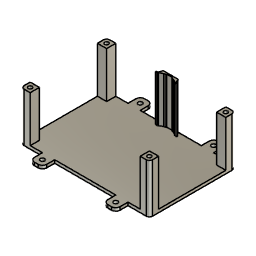
din_shelf_mount_2 v2 (Autodesk Fusion 360 design; units mm, degrees)
Autodesk Fusion 360 part; units mm, degrees
sketch "Sketch1" plane through (0, 0, 0) normal (0, 0, 1) x (1, 0, 0)
  line L0 (0, 0) -> (210, 0)
  line L1 (210, 0) -> (210, 140)
  line L2 (210, 140) -> (0, 140)
  line L3 (0, 140) -> (0, 0)
  line L4 (35, 140) -> (55, 140)
  line L5 (55, 140) -> (55, 153)
  line L6 (48, 160) -> (42, 160)
  line L7 (35, 153) -> (35, 140)
  line L8 (0, 70) -> (210, 70)
  line L9 (105, 140) -> (105, 0)
  circle A0 centre (45, 150) radius 3.5
  arc A1 (42, 160) -> (35, 153) centre (42, 153) ccw
  arc A2 (55, 153) -> (48, 160) centre (48, 153) ccw
  arc A3 (35, -13) -> (42, -20) centre (42, -13) ccw
  line L10 (48, -20) -> (42, -20)
  circle A4 centre (45, -10) radius 3.5
  arc A5 (48, -20) -> (55, -13) centre (48, -13) ccw
  line L11 (35, -13) -> (35, 0)
  line L12 (55, 0) -> (55, -13)
  arc A6 (162, 160) -> (155, 153) centre (162, 153) ccw
  arc A7 (175, 153) -> (168, 160) centre (168, 153) ccw
  line L13 (162, 160) -> (168, 160)
  circle A8 centre (165, 150) radius 3.5
  line L14 (175, 153) -> (175, 140)
  line L15 (155, 140) -> (155, 153)
  arc A9 (155, -13) -> (162, -20) centre (162, -13) ccw
  circle A10 centre (165, -10) radius 3.5
  line L16 (162, -20) -> (168, -20)
  arc A11 (168, -20) -> (175, -13) centre (168, -13) ccw
  line L17 (155, 0) -> (155, -13)
  line L18 (175, -13) -> (175, 0)
  point P0 (35, 160)
  point P1 (35, -20)
  point P2 (175, 160)
  point P3 (175, -20)
  dimension "d1" = 210
  dimension "d2" = 140
  dimension "d3" = 20
  dimension "d4" = 20
  dimension "d5" = 35
  dimension "d6" = 7
  dimension "d7" = 10
  dimension "d8" = 10
  dimension "d9" = 7
  constraint horizontal L0
  constraint vertical L1
  constraint horizontal L2
  constraint vertical L3
  constraint coincident L0.start L3.end
  constraint horizontal L4
  constraint vertical L5
  constraint horizontal L6
  constraint vertical L7
  constraint coincident L2 L4.start
  constraint midpoint L3 L8.start
  constraint midpoint L1 L8.end
  constraint midpoint L2 L9.start
  constraint midpoint L0 L9.end
  constraint coincident P0 L6
  constraint coincident P0 L7
  constraint tangent L6 A1
  constraint tangent L7 A1
  constraint tangent L5 A2
  constraint tangent L6 A2
  constraint equal A1 A2
  constraint symmetric L4.start L8 L11.end
  constraint symmetric L4.end L8 L12.start
  constraint symmetric P0 L8 P1
  constraint symmetric L8 A0 A4
  constraint symmetric L8 L6.end A3.end
  constraint symmetric L8 L7.start A3.start
  constraint symmetric L8 A1 A3
  constraint symmetric L8 L5.end A5.end
  constraint symmetric L8 L6.start L10.start
  constraint symmetric L8 A2 A5
  constraint symmetric L4.start L9 L14.end
  constraint symmetric L4.end L9 L15.start
  constraint symmetric P0 L9 P2
  constraint symmetric L9 A0 A8
  constraint symmetric L9 L6.end A7.end
  constraint symmetric L9 L7.start A7.start
  constraint symmetric L9 A1 A7
  constraint symmetric L9 L5.end A6.end
  constraint symmetric L9 L6.start A6.start
  constraint symmetric L9 A2 A6
  constraint symmetric L9 A3.start A11.end
  constraint symmetric L9 P1 P3
  constraint symmetric L9 L10.start A9.end
  constraint symmetric L9 A5.end A9.start
  constraint symmetric L9 A3.end L16.end
  constraint symmetric L9 A3 A11
  constraint symmetric L9 A4 A10
  constraint symmetric L9 A5 A9
  constraint symmetric L9 L11.end L18.end
  constraint symmetric L9 L12.start L17.start
  measures "d1" distance of L0.start L0.end
  measures "d2" distance of L0.start L2.end
  measures "d3" distance of L4.start L4.end
  measures "d4" distance of L4.start P0
  measures "d5" distance of L3 L7
  measures "d6" diameter of A0
  measures "d7" distance of L6 A0.centre
  measures "d8" distance of L7 A0.centre
  measures "d9" radius of A1
extrude "Extrude1" add sketch "Sketch1" along normal blind 5 makes body 1
sketch "Sketch2" plane through (0, 0, 5) normal (0, 0, 1) x (-1, 0, 0)
  circle A0 centre (-45, 10) radius 3.5
  circle A1 centre (-45, -150) radius 3.5
  circle A2 centre (-165, -150) radius 3.5
  circle A3 centre (-165, 10) radius 3.5
  line L0 (-55, 0) -> (-155, 0)
  line L1 (-155, 0) -> (-155, 13)
  arc A4 (-155, 13) -> (-162, 20) centre (-162, 13) ccw
  line L2 (-162, 20) -> (-168, 20)
  arc A5 (-168, 20) -> (-175, 13) centre (-168, 13) ccw
  line L3 (-175, 13) -> (-175, 0)
  line L4 (-175, 0) -> (-210, 0)
  line L5 (-210, 0) -> (-210, -140)
  line L6 (-210, -140) -> (-175, -140)
  line L7 (-175, -140) -> (-175, -153)
  arc A6 (-175, -153) -> (-168, -160) centre (-168, -153) ccw
  line L8 (-168, -160) -> (-162, -160)
  arc A7 (-162, -160) -> (-155, -153) centre (-162, -153) ccw
  line L9 (-155, -153) -> (-155, -140)
  line L10 (-155, -140) -> (-55, -140)
  line L11 (-55, -140) -> (-55, -153)
  arc A8 (-55, -153) -> (-48, -160) centre (-48, -153) ccw
  line L12 (-48, -160) -> (-42, -160)
  arc A9 (-42, -160) -> (-35, -153) centre (-42, -153) ccw
  line L13 (-35, -153) -> (-35, -140)
  line L14 (-35, -140) -> (0, -140)
  line L15 (0, -140) -> (0, 0)
  line L16 (0, 0) -> (-35, 0)
  line L17 (-35, 0) -> (-35, 13)
  arc A10 (-35, 13) -> (-42, 20) centre (-42, 13) ccw
  line L18 (-42, 20) -> (-48, 20)
  arc A11 (-48, 20) -> (-55, 13) centre (-48, 13) ccw
  line L19 (-55, 13) -> (-55, 0)
  line L20 (0, -140) -> (-15, -140)
  line L21 (-15, -140) -> (-15, -125)
  line L22 (-15, -125) -> (0, -125)
  line L23 (0, -125) -> (0, -140)
  line L24 (-210, -140) -> (-195, -140)
  line L25 (-195, -140) -> (-195, -125)
  line L26 (-195, -125) -> (-210, -125)
  line L27 (-210, -125) -> (-210, -140)
  line L28 (0, 0) -> (-15, 0)
  line L29 (-15, 0) -> (-15, -15)
  line L30 (-15, -15) -> (0, -15)
  line L31 (0, -15) -> (0, 0)
  line L32 (-210, 0) -> (-195, 0)
  line L33 (-195, 0) -> (-195, -15)
  line L34 (-195, -15) -> (-210, -15)
  line L35 (-210, -15) -> (-210, 0)
  dimension "d12" = 15
  dimension "d13" = 15
  dimension "d14" = 15
  dimension "d15" = 15
  dimension "d16" = 15
  dimension "d17" = 15
  dimension "d18" = 15
  dimension "d19" = 15
  constraint horizontal L20
  constraint vertical L21
  constraint horizontal L22
  constraint vertical L23
  constraint coincident L14.end L15.start
  constraint horizontal L24
  constraint vertical L25
  constraint horizontal L26
  constraint vertical L27
  constraint coincident L5.end L6.start
  constraint horizontal L28
  constraint vertical L29
  constraint horizontal L30
  constraint vertical L31
  constraint coincident L15.end L16.start
  constraint horizontal L32
  constraint vertical L33
  constraint horizontal L34
  constraint vertical L35
  constraint coincident L4.end L5.start
  measures "d12" distance of L14.end L20.end
  measures "d13" distance of L14.end L22.end
  measures "d14" distance of L5.end L24.end
  measures "d15" distance of L5.end L26.end
  measures "d16" distance of L15.end L28.end
  measures "d17" distance of L15.end L30.end
  measures "d18" distance of L4.end L32.end
  measures "d19" distance of L4.end L34.end
extrude "Extrude2" add sketch "Sketch2" along normal blind 75 contours L15 L16 L28 L29 L30 L31 | L4 L5 L32 L33 L34 L35 | L14 L15 L20 L21 L22 L23 | L5 L6 L24 L25 L26 L27 bodies 1
fillet "Fillet1" radius 5 4 edges at (0, 140, 40) (0, 0, 40) (210, 140, 40) (210, 0, 40) on bodies 1
sketch "Sketch3" plane through (0, 0, 5) normal (0, 0, 1) x (-1, 0, 0)
  line L0 (-15, -15) -> (-15, 0)
  line L1 (-15, 0) -> (-35, 0)
  line L2 (-35, 0) -> (-35, 13)
  arc A0 (-35, 13) -> (-42, 20) centre (-42, 13) ccw
  line L3 (-42, 20) -> (-48, 20)
  arc A1 (-48, 20) -> (-55, 13) centre (-48, 13) ccw
  line L4 (-55, 13) -> (-55, 0)
  line L5 (-55, 0) -> (-155, 0)
  line L6 (-155, 0) -> (-155, 13)
  arc A2 (-155, 13) -> (-162, 20) centre (-162, 13) ccw
  line L7 (-162, 20) -> (-168, 20)
  arc A3 (-168, 20) -> (-175, 13) centre (-168, 13) ccw
  line L8 (-175, 13) -> (-175, 0)
  line L9 (-175, 0) -> (-195, 0)
  line L10 (-195, 0) -> (-195, -15)
  line L11 (-195, -15) -> (-210, -15)
  line L12 (-210, -15) -> (-210, -125)
  line L13 (-210, -125) -> (-195, -125)
  line L14 (-195, -125) -> (-195, -140)
  line L15 (-195, -140) -> (-175, -140)
  line L16 (-175, -140) -> (-175, -153)
  arc A4 (-175, -153) -> (-168, -160) centre (-168, -153) ccw
  line L17 (-168, -160) -> (-162, -160)
  arc A5 (-162, -160) -> (-155, -153) centre (-162, -153) ccw
  line L18 (-155, -153) -> (-155, -140)
  line L19 (-155, -140) -> (-55, -140)
  line L20 (-55, -140) -> (-55, -153)
  arc A6 (-55, -153) -> (-48, -160) centre (-48, -153) ccw
  line L21 (-48, -160) -> (-42, -160)
  arc A7 (-42, -160) -> (-35, -153) centre (-42, -153) ccw
  line L22 (-35, -153) -> (-35, -140)
  line L23 (-35, -140) -> (-15, -140)
  line L24 (-15, -140) -> (-15, -125)
  line L25 (-15, -125) -> (0, -125)
  line L26 (0, -125) -> (0, -15)
  line L27 (0, -15) -> (-15, -15)
  circle A8 centre (-45, 10) radius 3.5
  circle A9 centre (-45, -150) radius 3.5
  circle A10 centre (-165, -150) radius 3.5
  circle A11 centre (-165, 10) radius 3.5
  line L28 (-116.5, -140) -> (-93.5, -140)
  line L29 (-87.5, -133.5) -> (-87.5, -132.5)
  arc A12 (-100.1064, -137.0284) -> (-100.5, -137.5169) centre (-100, -137.5169) ccw
  arc A13 (-90.5, -132.5) -> (-91.7987, -132.979) centre (-90.5, -134.5) ccw
  line L30 (-119.5, -132.5) -> (-122.5, -132.5)
  arc A14 (-88.5, -133.5) -> (-91.5, -136.5) centre (-88.5, -136.5) ccw
  arc A15 (-112.6132, -136.2584) -> (-112.4547, -136.3163) centre (-106.1884, -118.9099) ccw
  arc A16 (-97.3868, -136.2584) -> (-97.2095, -136.1954) centre (-105, -114.555) ccw
  line L31 (-112.4547, -136.3163) -> (-112.7905, -136.1954)
  arc A17 (-97.3868, -136.2584) -> (-91.7987, -132.979) centre (-103.8116, -118.9099) ccw
  arc A18 (-112.6132, -136.2584) -> (-109.8936, -137.0284) centre (-105, -114.555) ccw
  arc A19 (-118.5, -138) -> (-116.5, -140) centre (-116.5, -138) ccw
  line L32 (-122.5, -132.5) -> (-122.5, -133.5)
  line L33 (-109.5, -137.8785) -> (-109.5, -137.5169)
  arc A20 (-93.5, -140) -> (-91.5, -138) centre (-93.5, -138) ccw
  arc A21 (-118.5, -136.5) -> (-121.5, -133.5) centre (-121.5, -136.5) ccw
  line L34 (-118.5, -136.5) -> (-118.5, -138)
  line L35 (-91.5, -138) -> (-91.5, -136.5)
  line L36 (-87.5, -132.5) -> (-90.5, -132.5)
  line L37 (-122.5, -133.5) -> (-121.5, -133.5)
  line L38 (-100.5, -137.5169) -> (-100.5, -137.8785)
  arc A22 (-118.2013, -132.979) -> (-112.6132, -136.2584) centre (-106.1884, -118.9099) ccw
  arc A23 (-118.2013, -132.979) -> (-119.5, -132.5) centre (-119.5, -134.5) ccw
  line L39 (-97.2095, -136.1954) -> (-97.5453, -136.3163)
  line L40 (-88.5, -133.5) -> (-87.5, -133.5)
  arc A24 (-112.7905, -136.1954) -> (-112.6132, -136.2584) centre (-105, -114.555) ccw
  arc A25 (-97.5453, -136.3163) -> (-97.3868, -136.2584) centre (-103.8116, -118.9099) ccw
  line L41 (-100.5, -137.8785) -> (-109.5, -137.8785)
  arc A26 (-100.1064, -137.0284) -> (-97.3868, -136.2584) centre (-105, -114.555) ccw
  arc A27 (-109.5, -137.5169) -> (-109.8936, -137.0284) centre (-110, -137.5169) ccw
  point P0 (-105, -140)
extrude "Extrude3" add sketch "Sketch3" along normal blind 75 separate body contours L19 L28 L29 A12 A13 L30 A14 A17 A18 A19 L32 L33 A20 A21 L34 L35 L36 L37 L38 A22 A23 L40 L41 A26 A27 makes body 2
sketch "Sketch4" plane through (0, 0, 80) normal (0, 0, 1) x (-1, 0, 0)
  arc A0 (-5, -140) -> (0, -135) centre (-5, -135) ccw
  line L0 (0, -135) -> (0, -125)
  line L1 (0, -125) -> (-15, -125)
  line L2 (-15, -125) -> (-15, -140)
  line L3 (-15, -140) -> (-5, -140)
  circle A1 centre (-7.5, -132.5) radius 3.2
  circle A2 centre (-202.5, -132.5) radius 3.2
  line L4 (-205, -140) -> (-195, -140)
  line L5 (-195, -140) -> (-195, -125)
  circle A3 centre (-202.5, -7.5) radius 3.2
  line L6 (-210, -5) -> (-210, -15)
  line L7 (-210, -15) -> (-195, -15)
  circle A4 centre (-7.5, -7.5) radius 3.2
  line L8 (-15, -15) -> (0, -15)
  line L9 (-15, 0) -> (-15, -15)
  dimension "d26" = 6.4
  dimension "d27" = 7.5
  dimension "d28" = 7.5
  dimension "d29" = 6.4
  dimension "d30" = 7.5
  dimension "d31" = 7.5
  dimension "d32" = 6.4
  dimension "d33" = 7.5
  dimension "d34" = 7.5
  dimension "d35" = 6.4
  dimension "d36" = 7.5
  dimension "d37" = 7.5
  measures "d26" diameter of A1
  measures "d27" distance of L2 A1.centre
  measures "d28" distance of L1 A1.centre
  measures "d29" diameter of A2
  measures "d30" distance of A2.centre L4
  measures "d31" distance of A2.centre L5
  measures "d32" diameter of A3
  measures "d33" distance of A3.centre L6
  measures "d34" distance of A3.centre L7
  measures "d35" diameter of A4
  measures "d36" distance of A4.centre L8
  measures "d37" distance of A4.centre L9
extrude "Extrude4" cut sketch "Sketch4" against normal blind 9.5 contours A1 | A2 | A3 | A4 bodies 1
